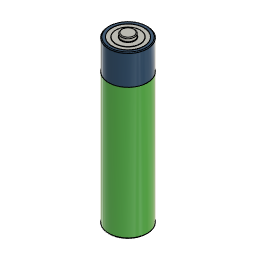
Battery (AAA) (Autodesk Fusion 360 design; units mm, degrees)
Autodesk Fusion 360 part; units mm, degrees
sketch "Base" plane through (0, 0, 0) normal (0, 0, 1) x (1, 0, 0) in component "Battery (AAA)"
  circle A0 centre (0, 0) radius 5.15
  constraint coincident A0.centre origin
extrude "Extrude1" add sketch "Base" along normal blind 43 in component "Battery (AAA)"
fillet "Fillet1" radius 0.3 1 edges at (-4.8015, -1.8623, 0) in component "Battery (AAA)"
fillet "Fillet3" radius 0.2 1 edges at (-4.8015, -1.8623, 43) in component "Battery (AAA)"
sketch "Bottom" plane through (0, 0, 0) normal (0, 0, -1) x (1, 0, 0) in component "Battery (AAA)"
  circle A0 centre (0, 0) radius 4.85
  circle A1 centre (0, 0) radius 3.25
  circle A2 centre (0, 0) radius 3
  constraint coincident A0.centre A1.centre
  constraint concentric A0 A2
extrude "Extrude2" cut sketch "Bottom" against normal blind 0.5 contours A1 in component "Battery (AAA)"
fillet "Fillet2" radius 0.2 1 edges at (-2.797, 1.0848, 0) in component "Battery (AAA)"
sketch "Top" plane through (0, 0, 43) normal (0, 0, 1) x (-1, 0, 0) in component "Battery (AAA)"
  circle A0 centre (0, 0) radius 4.95
  circle A1 centre (0, 0) radius 4.25
  circle A2 centre (0, 0) radius 3.25
  circle A3 centre (0, 0) radius 1.75
  constraint coincident A0.centre A1.centre
  constraint concentric A2 A3
extrude "Extrude3" cut sketch "Top" against normal blind 0.05 contours A1 in component "Battery (AAA)"
extrude "Extrude4" add sketch "Top" along normal blind 1 contours A3 in component "Battery (AAA)"
fillet "Fillet4" radius 0.05 1 edges at (3.0301, 1.1753, 43) in component "Battery (AAA)"
fillet "Fillet5" radius 0.2 1 edges at (1.6316, 0.6328, 44) in component "Battery (AAA)"
fillet "Fillet6" radius 0.1 1 edges at (1.6316, -0.6328, 43) in component "Battery (AAA)"
ref_plane "WorkPlane1" through (0, 0, 35) normal (0, 0, 1) x (1, 0, 0) in component "Battery (AAA)"
split_face "SplitFace1" 1 faces at (5.1436, -0.2567, 28.6333) by plane through (0, 0, 35) normal (0, 0, 1) in component "Battery (AAA)"
component "Battery (AAA)" placed x (1, 0, 0) y (0, 1, 0) z (0, 0, 1) at (0, 0, 0)
named bodies: "Battery (AAA)"
